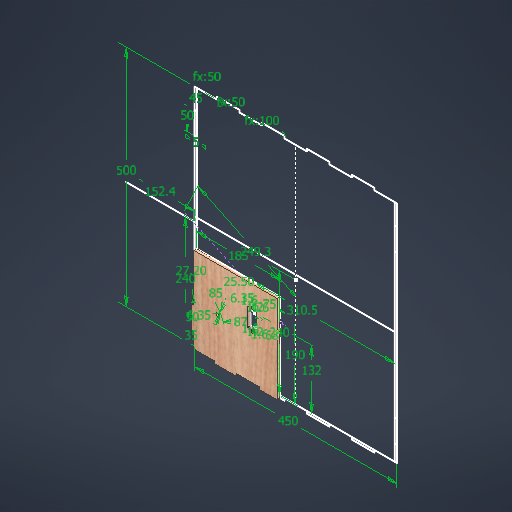
# Autodesk Inventor part: Cut Pegboard Panel Skiba
Saved by Autodesk Inventor 2026.2 (Build 302298000, 298)
## iProperties
Created: 2024-10-14
Part Number: Cut Pegboard Panel Skiba
Material: Wood (Birch)
Document SubType Name: Modeling
Designer: 239tr
Density: 0.55 g/cm^3
Appearance: Birch - Natural Polished
Author: 239tr
Autodesk Inventor part; units mm, degrees
ref_plane "YZ Plane" through (0, 0, 0) normal (1, 0, 0) x (0, 1, 0)
ref_plane "XZ Plane" through (0, 0, 0) normal (0, 1, 0) x (-1, 0, 0)
ref_plane "XY Plane" through (0, 0, 0) normal (0, 0, 1) x (1, 0, 0)
sketch "Block1" plane through (0, 0, 0) normal (0, 0, 1) x (1, 0, 0)
  circle A0 centre (-65.4812, 52.5391) radius 2.75 construction
  circle A1 centre (-65.4812, 52.5391) radius 5 construction
  line L0 (-55.4812, 62.5391) -> (-95.9812, 62.5391)
  line L1 (-95.9812, 62.5391) -> (-95.9812, 42.5391)
  arc A2 (-100.7311, 56.2391) -> (-100.7311, 58.8391) centre (-98.9812, 57.5391) ccw
  arc A3 (-100.7311, 46.2391) -> (-100.7311, 48.8391) centre (-98.9812, 47.5391) ccw
  line L2 (-95.9812, 42.5391) -> (-55.4812, 42.5391)
  arc A4 (-50.7312, 48.8391) -> (-50.7312, 46.2391) centre (-52.4812, 47.5391) ccw
  arc A5 (-50.7312, 58.8391) -> (-50.7312, 56.2391) centre (-52.4812, 57.5391) ccw
  line L3 (-55.4812, 62.5391) -> (-55.4812, 42.5391)
  point P0 (-74.5923, 52.5391)
sketch "open sketch to change param" plane through (0, 0, 0) normal (0, 0, 1) x (1, 0, 0)
  line L0 (0, 0) -> (450, 0)
  line L1 (450, 0) -> (450, 500)
  line L2 (0, 500) -> (0, 0)
  line L3 (225, 500) -> (225, 0) construction
  line L4 (0, 455) -> (5, 455)
  line L5 (5, 455) -> (5, 405)
  line L6 (5, 405) -> (0, 405)
  line L7 (0, 405) -> (0, 455)
  line L8 (450, 405) -> (450, 455)
  line L9 (100, 500) -> (100, 505)
  line L10 (100, 505) -> (50, 505)
  line L11 (50, 505) -> (50, 500)
  line L12 (50, 500) -> (0, 500)
  line L13 (200, 500) -> (200, 505)
  line L14 (200, 505) -> (150, 505)
  line L15 (150, 505) -> (150, 500)
  line L16 (300, 500) -> (300, 505)
  line L17 (300, 505) -> (250, 505)
  line L18 (250, 505) -> (250, 500)
  line L19 (400, 500) -> (400, 505)
  line L20 (400, 505) -> (350, 505)
  line L21 (350, 505) -> (350, 500)
  line L22 (150, 500) -> (100, 500)
  line L23 (250, 500) -> (200, 500)
  line L24 (450, 500) -> (400, 500)
  line L25 (350, 500) -> (300, 500)
  line L26 (5, 500) -> (5, 0)
  line L27 (445, 500) -> (445, 0)
  line L28 (0, 85) -> (5, 85)
  line L29 (0, 35) -> (5, 35)
  line L30 (450, 455) -> (445, 455)
  line L31 (445, 405) -> (450, 405)
  line L32 (450, 85) -> (445, 85)
  line L33 (450, 35) -> (445, 35)
  line L34 (0, 250) -> (445, 250)
  line L35 (100, 0) -> (100, -5)
  line L36 (100, -5) -> (50, -5)
  line L37 (50, -5) -> (50, 0)
  line L38 (200, 0) -> (200, -5)
  line L39 (200, -5) -> (150, -5)
  line L40 (150, -5) -> (150, 0)
  line L41 (300, 0) -> (300, -5)
  line L42 (300, -5) -> (250, -5)
  line L43 (250, -5) -> (250, 0)
  line L44 (400, 0) -> (400, -5)
  line L45 (400, -5) -> (350, -5)
  line L46 (350, -5) -> (350, 0)
  circle A0 centre (134.5, 132) radius 3.175
  line L47 (134.5, 132) -> (201.9264, 140.8134) construction
  line L48 (201.9264, 140.8134) -> (126.9265, 140.7316) construction
  line L49 (126.9265, 140.7316) -> (57.1208, 92.2325) construction
  line L50 (134.5, 132) -> (57.1208, 92.2325) construction
  line L51 (134.5, 132) -> (5, 132) construction
  circle A1 centre (57.1208, 92.2325) radius 3.175
  circle A2 centre (139.5, 145) radius 2.18
  circle A3 centre (129.5, 145) radius 2.18
  circle A4 centre (139.5, 98.5) radius 2.18
  circle A5 centre (129.5, 98.5) radius 2.18
  line L52 (201.9264, 140.8134) -> (-23.205, 247.8943) construction
  line L53 (133.9, 148) -> (133.9, 142)
  line L54 (133.9, 148) -> (135.1, 148)
  line L55 (135.1, 142) -> (135.1, 148)
  line L56 (133.9, 142) -> (135.1, 142)
  line L57 (135.1, 101.5) -> (133.9, 101.5)
  line L58 (133.9, 101.5) -> (133.9, 95.5)
  line L59 (133.9, 95.5) -> (135.1, 95.5)
  line L60 (135.1, 95.5) -> (135.1, 101.5)
  circle A6 centre (129.5, 145) radius 0.8
  circle A7 centre (139.5, 145) radius 0.8
  circle A8 centre (129.5, 98.5) radius 0.8
  circle A9 centre (139.5, 98.5) radius 0.8
  line L61 (0, 0) -> (0, 240)
  line L62 (0, 240) -> (-152.4, 240)
  line L63 (5, 0) -> (190, 0)
  line L64 (190, 0) -> (190, 190)
  line L65 (190, 190) -> (5, 190)
  line L66 (5, 190) -> (5, 0)
  circle A10 centre (134.5, 132) radius 2.75 construction
  circle A11 centre (134.5, 132) radius 5 construction
  line L67 (124.5, 142) -> (124.5, 101.5)
  line L68 (124.5, 101.5) -> (144.5, 101.5)
  arc A12 (130.8, 96.75) -> (128.2, 96.75) centre (129.5, 98.5) ccw
  arc A13 (140.8, 96.75) -> (138.2, 96.75) centre (139.5, 98.5) ccw
  line L69 (144.5, 101.5) -> (144.5, 142)
  arc A14 (138.2, 146.75) -> (140.8, 146.75) centre (139.5, 145) ccw
  arc A15 (128.2, 146.75) -> (130.8, 146.75) centre (129.5, 145) ccw
  line L70 (124.5, 142) -> (144.5, 142)
  point P0 (225, 240)
  point P1 (5, 480)
  point P2 (0, 455)
  point P3 (0, 405)
  point P4 (5, 405)
  point P5 (450, 35)
  point P6 (450, 85)
  point P7 (445, 85)
  point P8 (445, 405)
  point P9 (450, 405)
  point P10 (445, 35)
  point P11 (100, 0)
  point P12 (50, 0)
  point P13 (200, 0)
  point P14 (150, 0)
  point P15 (300, 0)
  point P16 (250, 0)
  point P17 (400, 0)
  point P18 (350, 0)
  point P19 (138.2, 146.75)
  point P20 (140.8, 146.75)
  point P21 (128.2, 146.75)
  point P22 (130.8, 146.75)
  point P23 (140.8, 96.75)
  point P24 (138.2, 96.75)
  point P25 (130.8, 96.75)
  point P26 (128.2, 96.75)
  point P27 (134.5, 142)
  point P28 (134.5, 142)
  point P29 (134.5, 101.5)
  point P30 (134.5, 101.5)
  point P31 (135.1, 101.5)
  point P32 (133.9, 101.5)
  dimension "d4" = 240
  dimension "d5" = 50
  dimension "d6" = 5
  dimension "d17" = 50
  dimension "d18" = 50
  dimension "d28" = 100
  dimension "d33" = 500
  dimension "d34" = 5
  dimension "d35" = 45
  dimension "d83" = 50
  dimension "d84" = 35
  dimension "d100" = 450
  dimension "d101" = 6.35
  dimension "d102" = 310.5
  dimension "d103" = 132
  dimension "d104" = -27.2
  dimension "d105" = 87
  dimension "d106" = 68
  dimension "d107" = 75
  dimension "d108" = 85
  dimension "d111" = 6.35
  dimension "d122" = 249.3
  dimension "d123" = 25.5
  dimension "d125" = 6
  dimension "d127" = 1.2
  dimension "d128" = 6
  dimension "d129" = 1.2
  dimension "d130" = 1.6
  dimension "d131" = 1.6
  dimension "d132" = 1.6
  dimension "d133" = 1.6
  dimension "d134" = 240
  dimension "d135" = 152.4
  dimension "d136" = 185
  dimension "d137" = 190
  constraints: 134 end point, 24 symmetric about line, 14 parallel, 13 point on line, 12 perpendicular, 10 centre point, 7 coincident, 6 horizontal, 6 midpoint, 2 vertical, 1 collinear, 33 other
  measures "d4" distance from line of L0 point (225, 240)
  measures "d5" distance of L4.end L5.end
  measures "d6" distance of L5.end L6.end
  measures "d17" distance of L9.end L10.end
  measures "d18" distance between parallel lines of L2 L11
  measures "d28" distance of L9.end L13.end
  measures "d33" distance between parallel lines of L0 L12
  measures "d34" distance between parallel lines of L12 L10
  measures "d35" distance between parallel lines of L4 L12
  measures "d83" distance between parallel lines of L29 L28
  measures "d84" distance between parallel lines of L0 L29
  measures "d100" distance between parallel lines of L2 L1
  measures "d101" diameter of A0
  measures "d102" distance from line of L47.start L27
  measures "d103" distance from line of L0 L47.start
  measures "d104" angle of L51 L50
  measures "d105" distance of L47.start L49.end
  measures "d106" distance of L47.start L47.end
  measures "d107" distance of L47.end L48.end
  measures "d108" distance of L48.end L49.end
  measures "d111" diameter of A1
  measures "d122" distance of L47.end L52.end
  measures "d123" angle of L48 L52
  measures "d125" distance of L56.end L55.end
  measures "d127" distance of L56.start L56.end
  measures "d128" distance of L59.end L57.start
  measures "d129" distance between parallel lines of L58 L60
  measures "d130" diameter of A6
  measures "d131" diameter of A7
  measures "d132" diameter of A8
  measures "d133" diameter of A9
  measures "d134" distance of L0.start L61.end
  measures "d135" distance of L61.end L62.end
  measures "d136" distance of L65.end L64.end
  measures "d137" distance of L64.end L63.end
extrude "Extrusion1" add sketch "open sketch to change param" along normal blind 6.35 contours L26 L65 L64 L0 | L2 L28 L26 L29 | L0 L35 L36 L37 | L0 L38 L39 L40 | L26 L34 L27 L0 L64 L65 | L26 L5 L12 L11 L10 L9 L22 L15 L14 L13 L23 L18 L17 L16 L25 L21 L20 L19 L24 L27 L34 | L2 L4 L5 L6 | L0 L41 L42 L43 | L27 L30 L1 L31 | L32 L1 L33 L27 | L0 L44 L45 L46 | A2 | A3 | A4 | A5
sketch "Sketch2" plane through (0, 0, 6.35) normal (0, 0, 1) x (1, 0, 0)
  line L0 (0, 0) -> (0, -5)
  line L1 (0, -5) -> (190, -5)
  line L2 (190, -5) -> (190, 190)
  line L3 (190, 190) -> (0, 190)
  line L4 (0, 190) -> (0, -5)
  line L5 (0, 190) -> (0, 568.7197)
  line L6 (5, 405) -> (5, 85) projected
  line L7 (0, 568.7197) -> (531.5547, 568.7197)
  line L8 (531.5547, 568.7197) -> (531.5547, -5)
  line L9 (531.5547, -5) -> (190, -5)
  dimension "d138" = 5
  dimension "d139" = 190
  dimension "d140" = 195
  constraints: 18 end point, 4 perpendicular, 3 parallel, 1 horizontal, 1 vertical
  measures "d138" distance of L0.start L0.end
  measures "d139" distance of L3.end L2.end
  measures "d140" distance of L2.end L1.end
extrude "Extrusion3" cut sketch "Sketch2" against normal blind 6.35 contours L5 L7 L8 L9 L2 L3
body "Solid1"
